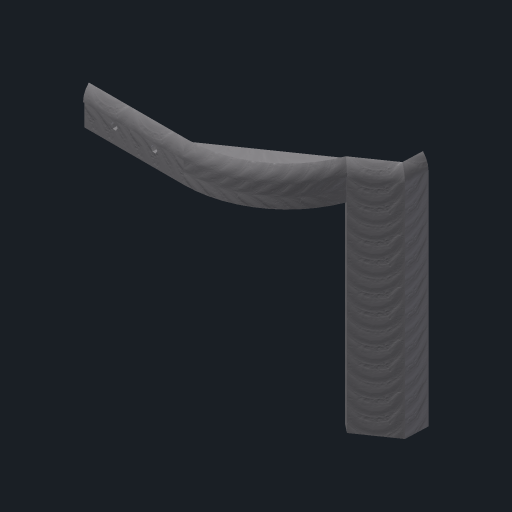
# Autodesk Inventor part: ESQUINA_REDONDEADA_R20
Saved by Autodesk Inventor 2024.3 (Build 283343000, 343)
## iProperties
Created: 2024-05-19
Part Number: ESQUINA_REDONDEADA_R20
Material: Steel, Mild, Welded
Document SubType Name: Modeling
Designer: Niler
Density: 7.85 g/cm^3
Appearance: Weld - Steel Mild
Author: Niler
Autodesk Inventor part; units mm, degrees
ref_plane "YZ Plane" through (0, 0, 0) normal (1, 0, 0) x (0, 1, 0)
ref_plane "XZ Plane" through (0, 0, 0) normal (0, 1, 0) x (-1, 0, 0)
ref_plane "XY Plane" through (0, 0, 0) normal (0, 0, 1) x (1, 0, 0)
sketch "Sketch1" plane through (0, 0, 0) normal (1, 0, 0) x (0, 1, 0)
  circle A0 centre (0, 0) radius 20
  line L0 (8.5, 8.5) -> (-16.9, 8.5)
  line L1 (8.5, 8.5) -> (8.5, -16.9)
  line L2 (0, 0) -> (0, 20)
  line L3 (0, 20) -> (-60.9241, 20)
  line L4 (-60.9241, 20) -> (-60.9241, 18.5)
  line L5 (-60.9241, 18.5) -> (0, 18.5)
  line L6 (0, 18.5) -> (0, 20)
  line L7 (0, 0) -> (14.1421, 14.1421)
  line L8 (0, 0) -> (20, 0)
  line L9 (-16.9, 8.5) -> (-16.9, 18.5)
  line L10 (-16.9, 8.5) -> (-22.9, 14.5)
  line L11 (-22.9, 14.5) -> (-22.9, 18.5)
  line L12 (12.3744, 12.3744) -> (12.1502, 13.2109)
  line L13 (11.3137, 13.435) -> (9.2071, 11.3284)
  line L14 (9.4313, 10.4919) -> (10.2678, 10.2678)
  line L15 (8.5, 8.5) -> (8.5, -16.9)
  line L16 (20, 0) -> (20, -60.9241)
  line L17 (20, -60.9241) -> (18.5, -60.9241)
  line L18 (18.5, -60.9241) -> (18.5, 0)
  line L19 (8.5, -16.9) -> (18.5, -16.9)
  line L20 (8.5, -16.9) -> (14.5, -22.9)
  line L21 (14.5, -22.9) -> (18.5, -22.9)
  arc A1 (9.2071, 11.3284) -> (9.4313, 10.4919) centre (9.5607, 10.9749) ccw
  arc A2 (12.1502, 13.2109) -> (11.3137, 13.435) centre (11.6673, 13.0815) ccw
  line L22 (10.4311, 10.4311) -> (9.483, 10.6851)
  arc A3 (9.3485, 11.187) -> (9.483, 10.6851) centre (9.5607, 10.9749) ccw
  line L23 (9.3485, 11.187) -> (11.4551, 13.2936)
  arc A4 (11.957, 13.1591) -> (11.4551, 13.2936) centre (11.6673, 13.0815) ccw
  line L24 (11.957, 13.1591) -> (12.2111, 12.2111)
  point P0 (0, 8.5)
  point P1 (-17.7041, 9.3041)
  point P2 (-16.9, 10.6953)
  dimension "d0" = 40
  dimension "d1" = 25.4
  dimension "d2" = 1.5
  dimension "d4" = 45
  dimension "d6" = 45
  dimension "d7" = 4
  dimension "d8" = 10
  dimension "d10" = 2.5
  dimension "d11" = 2.5
  dimension "d12" = 60
  dimension "d13" = 1.5
  dimension "d15" = 0.5
  dimension "d16" = 0.2
  constraints: 50 end point, 11 point on circle, 10 point on line, 6 symmetric about line, 5 centre point, 4 perpendicular, 4 tangent, 3 parallel, 2 equal length, 2 horizontal, 2 vertical, 1 coincident, 1 equal radius, 1 vertical alignment, 4 other
  measures "d0" diameter of A0
  measures "d1" distance of L0.start L1.end
  measures "d2" distance of L4.end L3.end
  measures "d4" angle of L2 L7
  measures "d6" angle of L9 L10
  measures "d7" distance of L10.end L11.end
  measures "d8" distance between parallel lines of L0 L5
  measures "d10" distance of L7.end L12.start
  measures "d11" distance of L0.start L14.end
  measures "d12" angle of L7 L12
  measures "d13" distance between parallel lines of L7 L13
  measures "d15" radius of A1
  measures "d16" distance between parallel lines of L13 L23
extrude "Extrusion1" add sketch "Sketch1" along normal blind 100 contours L7 L12 A2 L13 A1 L14 L0 L2 A0 | L7 L24 A4 L23 A3 L22 L14 A1 L13 A2 L12 | L5 L2 L0 L9 A0 | A0 L9 L5 | L7 L22 A3 L23 A4 L24 | L9 L10 A0 | A0 L10 L11 L5 L9
sketch "Sketch2" plane through (0, -22.9, 18.5) normal (0, 0, 1) x (1, 0, 0)
  line L0 (0, 22.9) -> (0, 0) projected
  line L1 (0, 0) -> (100, 0) projected
  line L2 (100, 22.9) -> (100, 0) projected
  line L3 (0, 22.9) -> (100, 22.9) projected
  line L4 (28.3257, 13.1) -> (26.6514, 16)
  line L5 (26.6514, 16) -> (28.3257, 18.9)
  line L6 (28.3257, 18.9) -> (31.6743, 18.9)
  line L7 (31.6743, 18.9) -> (33.3486, 16)
  line L8 (33.3486, 16) -> (31.6743, 13.1)
  line L9 (31.6743, 13.1) -> (28.3257, 13.1)
  line L10 (0, 6) -> (100, 6) projected
  circle A0 centre (30, 16) radius 1.65
  dimension "d20" = 10
  dimension "d21" = 5.8
  dimension "d22" = 30
  dimension "d25" = 3.3
  constraints: 12 end point, 1 centre point, 1 coincident, 1 horizontal alignment, 13 other
  measures "d20" distance from line of L10 point (30, 16)
  measures "d21" distance between parallel lines of L9 L6
  measures "d22" distance from line of point (30, 16) L0
  measures "d25" diameter of A0
extrude "Extrusion2" cut sketch "Sketch2" against normal blind 6 contours L4 L5 L6 L7 L8 L9 | A0
extrude "Extrusion3" cut sketch "Sketch2" against normal through all contours A0
sketch "Sketch3" plane through (0, -22.9, 18.5) normal (0, 0, 1) x (1, 0, 0)
  line L0 (0, 37.0421) -> (100, 37.0421) projected
  line L1 (0, 0) -> (100, 0) projected
  line L2 (0, 22.9) -> (0, 0) projected
  line L3 (0, 22.9) -> (0, 37.0421) projected
  line L4 (2.4384, 37.0421) -> (17.8575, 0)
  line L5 (0, 0) -> (100, 0) projected
  line L6 (2.4384, 37.0421) -> (0, 42.9) projected
  point P0 (0, 26.9698)
  dimension "d28" = 112.6
  constraints: 2 end point, 1 point on line
  measures "d28" angle of L4 L0
sketch "Sketch4" plane through (100, 14.1421, 14.1421) normal (0, 0.7071068, -0.7071068) x (-1, 0, 0)
  line L0 (100, 0) -> (0, 0) projected
  line L1 (0, -7.9792) -> (0, 0) projected
  line L2 (100, -7.9792) -> (0, -7.9792) projected
  circle A0 centre (80, -4) radius 1.5
  line L3 (100, -7.9792) -> (100, 0) projected
  line L4 (50, -7.9792) -> (50, 0)
  ellipse E0 centre (70, -18.8686) end of major axis (68.35, -18.8686) minor radius 1.1667 projected
  point P0 (100, -20)
  dimension "d34" = 3
  dimension "d35" = 4
  dimension "d46" = 20
  constraints: 2 end point, 2 midpoint, 1 centre point, 1 other
  measures "d34" diameter of A0
  measures "d35" distance from line of L0 A0.centre
  measures "d46" distance from line of L3 A0.centre
extrude "Extrusion5" cut sketch "Sketch4" against normal blind 3 contours A0
ref_plane "Work Plane1" through (50, 0, 0) normal (-1, 0, 0) x (0, 0, 1)
mirror "Mirror1" about plane through (50, 0, 0) normal (-1, 0, 0) of "Extrusion5", "Extrusion2", "Extrusion3"
sketch "Sketch5" plane through (0, 0, 0) normal (0, 1, 0) x (-1, 0, 0)
  line L0 (-100, 14.1421) -> (-227.2781, -74.3185) construction
  arc A0 (-100, 14.1421) -> (-193.7282, -51.0007) centre (-100, -85.8579) ccw
  line L1 (-193.7282, -51.0007) -> (-227.2781, -74.3185)
  line L2 (0, 14.1421) -> (-100, 14.1421) projected
  line L3 (-227.2781, -74.3185) -> (-228.0459, -94.3037)
  point P0 (0, 0)
  dimension "d49" = 155
  dimension "d50" = 100
  dimension "d57" = 145.2
  dimension "d58" = 20
  dimension "d59" = 127
  constraints: 6 end point, 2 point on circle, 1 centre point, 1 collinear, 1 point on line, 1 tangent
  measures "d49" distance of L0.start L0.end
  measures "d50" radius of A0
  measures "d57" angle of L0 L2
  measures "d58" distance of L0.end L3.end
  measures "d59" angle of L3 L0
sketch "Sketch6" plane through (100, 0, 0) normal (1, 0, 0) x (0, 0, -1)
  line L0 (-14.5, -22.9) -> (-8.5, -16.9) projected
  line L1 (-8.5, -16.9) -> (-8.5, 8.5) projected
  line L2 (-8.5, 8.5) -> (-14.1421, 14.1421) projected
  arc A0 (-14.1421, 14.1421) -> (-20, 0) centre (0, 0) ccw projected
  line L3 (-20, 0) -> (-18.5, 0) projected
  line L4 (-18.5, 0) -> (-18.5, -22.9) projected
  line L5 (-18.5, -22.9) -> (-14.5, -22.9) projected
sweep "Sweep1" add profiles "Sketch6" path "Sketch5" path curves A0 L1 L3
sketch "Sketch7" plane through (0, 0, 0) normal (0, 1, 0) x (-1, 0, 0)
  arc A0 (-100, 8.5) -> (-188.4399, -52.9674) centre (-100, -85.8579) ccw projected
  line L0 (-189.0563, -54.6246) -> (-221.7481, -77.346) projected
  line L1 (0, 8.5) -> (-100, 8.5) projected
  line L2 (-189.0563, -54.6246) -> (-98.2319, 8.5)
  line L3 (-188.4399, -52.9674) -> (-189.0563, -54.6246) projected
  point P0 (0, 0)
  point P1 (-224.0581, -78.9515)
  constraints: 2 end point, 1 collinear, 1 point on line
extrude "Extrusion6" add sketch "Sketch7" along normal blind 8.5 and the other way blind 16.9
sketch "Sketch8" plane through (0, 0, 18.5) normal (0, -1, 0) x (1, 0, 0)
  line L0 (0, 1.5) -> (0, 0) projected
  line L1 (0, 0) -> (100, 0) projected
  arc A0 (197.3236, -66.6925) -> (100, 0) centre (100, -104.3579) ccw projected
  line L2 (197.3236, -66.6925) -> (231.5494, -90.48) projected
  line L3 (231.5494, -90.48) -> (232.4005, -112.6364) projected
  line L4 (233.8994, -112.5789) -> (232.4005, -112.6364) projected
  line L5 (233.0196, -89.6751) -> (233.8994, -112.5789) projected
  line L6 (198.5553, -65.7218) -> (233.0196, -89.6751) projected
  arc A1 (198.5553, -65.7218) -> (100, 1.5) centre (100, -104.3579) ccw projected
  line L7 (0, 1.5) -> (100, 1.5) projected
  line L8 (197.3236, -66.6925) -> (231.5494, -90.48) projected
  line L9 (197.3236, -66.6925) -> (198.5553, -65.7218)
  point P0 (0, -18.5)
  constraints: 2 end point
extrude "Extrusion7" add sketch "Sketch8" along normal up to surface (22.9 mm away) contours L6 L5 L4 L3 L2 L9
sketch "Sketch9" plane through (0, -22.9, 14.5) normal (0, -1, 0) x (1, 0, 0)
  line L0 (0, 4) -> (0, 0) projected
  line L1 (0, 0) -> (100, 0) projected
  arc A0 (194.0244, -65.2707) -> (100, 0) centre (100, -100.3579) ccw projected
  line L2 (227.6289, -88.6264) -> (194.0244, -65.2707) projected
  line L3 (227.6289, -88.6264) -> (228.4035, -108.79) projected
  line L4 (233.8994, -108.5789) -> (228.4035, -108.79) projected
  line L5 (233.0196, -85.6751) -> (233.8994, -108.5789) projected
  line L6 (198.5553, -61.7218) -> (233.0196, -85.6751) projected
  line L7 (197.3236, -62.6925) -> (198.5553, -61.7218) projected
  arc A1 (197.3236, -62.6925) -> (100, 4) centre (100, -100.3579) ccw projected
  line L8 (0, 4) -> (100, 4) projected
  line L9 (197.3236, -62.6925) -> (194.0244, -65.2707)
  line L10 (221.7481, -91.846) -> (227.6289, -88.6264) projected
  line L11 (221.7481, -91.846) -> (222.4079, -109.0203) projected
  line L12 (228.4035, -108.79) -> (222.4079, -109.0203) projected
  line L13 (227.6289, -88.6264) -> (228.4035, -108.79) projected
  line L14 (227.6289, -88.6264) -> (194.0244, -65.2707) projected
  spline S0 degree 7 poles (194.0244, -65.2707) (193.9847, -65.3016) (193.945, -65.3324) (193.9053, -65.3633) (193.8655, -65.3941) (193.8258, -65.425) (193.786, -65.4558) (193.7437, -65.4886) (193.7411, -65.4906) (193.7385, -65.4926) (193.736, -65.4946) (193.7334, -65.4966) (193.7308, -65.4987) (193.7282, -65.5007) knots 0 0 0 0 0 0 0 0 0.938902 0.938902 0.938902 0.938902 0.938902 0.938902 1 1 1 1 1 1 1 1 projected
  line L15 (189.0563, -69.1246) -> (193.7282, -65.5007) projected
  line L16 (221.7481, -91.846) -> (189.0563, -69.1246) projected
  line L17 (221.7481, -91.846) -> (227.6289, -88.6264) projected
  point P0 (0, -14.5)
  point P1 (221.7481, -91.846)
  constraints: 2 end point, 1 other
extrude "Extrusion8" add sketch "Sketch9" along normal blind 200 contours L7 L6 L5 L4 L3 L2 L9 | L2 L10 L16 L15 S0 | L3 L12 L11 L10
sketch "Sketch10" plane through (0, -22.9, 14.5) normal (0, 1, 0) x (1, 0, 0)
  line L0 (-25.5463, 168.5365) -> (280.7905, 168.5365)
  line L1 (280.7905, 168.5365) -> (280.7905, -16.8779)
  line L2 (280.7905, -16.8779) -> (-25.5463, -16.8779)
  line L3 (-25.5463, -16.8779) -> (-25.5463, 168.5365)
  point P0 (0, 14.5)
  constraints: 8 end point, 2 parallel, 1 horizontal, 1 perpendicular
body "Solid1"
